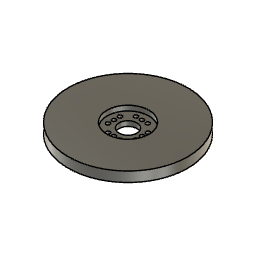
Rueda (Autodesk Fusion 360 design; units mm, degrees)
Autodesk Fusion 360 part; units mm, degrees
sketch "Sketch1" plane through (0, 0, 0) normal (0, 0, 1) x (1, 0, 0)
  circle A0 centre (0, 0) radius 30
  circle A1 centre (0, 0) radius 4.5
  line L0 (7, -7) -> (-7, -7)
  line L1 (-7, -7) -> (-7, 7)
  line L2 (-7, 7) -> (7, 7)
  line L3 (7, 7) -> (7, -7)
  line L4 (7, -7) -> (-7, 7) construction
  line L5 (-7, -7) -> (7, 7) construction
  line L6 (7, 0) -> (7, 4)
  line L7 (7, 0) -> (7, -4)
  circle A2 centre (7, 3) radius 1
  circle A3 centre (7, 0) radius 1
  circle A4 centre (7, -3) radius 1
  circle A5 centre (-3, 7) radius 1
  circle A6 centre (0, 7) radius 1
  circle A7 centre (3, 7) radius 1
  circle A8 centre (-7, -3) radius 1
  circle A9 centre (-7, 0) radius 1
  circle A10 centre (-7, 3) radius 1
  circle A11 centre (3, -7) radius 1
  circle A12 centre (0, -7) radius 1
  circle A13 centre (-3, -7) radius 1
  dimension "d1" = 60
  dimension "d2" = 9
  dimension "d3" = 14
  dimension "d4" = 14
  dimension "d5" = 4
  dimension "d6" = 4
  dimension "d7" = 2
  dimension "d8" = 2
  dimension "d11" = 0
  dimension "d12" = 0
  dimension "d14" = 360
  constraint coincident A0.centre A1.centre
  constraint concentric A0 A1
  constraint horizontal L0
  constraint perpendicular L0 L1
  constraint parallel L0 L2
  constraint parallel L1 L3
  constraint coincident L4 A0.centre
  constraint coincident L5 A0.centre
  constraint midpoint L3 L6.start
  constraint parallel L3 L6
  constraint parallel L3 L7
  constraint coincident L6.end A2
  constraint coincident L6.start L7.start
  constraint coincident L7.end A4
  measures "d1" diameter of A0
  measures "d2" diameter of A1
  measures "d3" distance of L1.end L2.end
  measures "d4" distance of L0.end L1.end
  measures "d5" distance of L6.start L6.end
  measures "d6" distance of L6.start L7.end
  measures "d7" diameter of A2
  measures "d8" diameter of A3
extrude "Extrude1" add sketch "Sketch1" along normal blind 5 contours A0 | L0 L1 L2 L3 L6 L7 A2 A3 A4 A5 A6 A7 A8 A9 A10 A11 A12 A13
sketch "Sketch2" plane through (0, 0, 5) normal (0, 0, 1) x (-1, 0, 0)
  circle A0 centre (-7, 3) radius 1
  circle A1 centre (3, 7) radius 1
  circle A2 centre (0, 7) radius 1
  circle A3 centre (0, -7) radius 1
  circle A4 centre (-3, 7) radius 1
  circle A5 centre (3, -7) radius 1
  circle A6 centre (0, 0) radius 4.5
  circle A7 centre (-7, -3) radius 1
  circle A8 centre (-7, 0) radius 1
  circle A9 centre (7, 0) radius 1
  circle A10 centre (-3, -7) radius 1
  circle A11 centre (7, -3) radius 1
  circle A12 centre (7, 3) radius 1
  circle A13 centre (0, 0) radius 30
  circle A14 centre (0, 0) radius 10.5
  dimension "d17" = 21
  constraint coincident A6.centre A13.centre
  measures "d17" diameter of A14
extrude "Extrude2" cut sketch "Sketch2" against normal blind 2.5 contours A14
